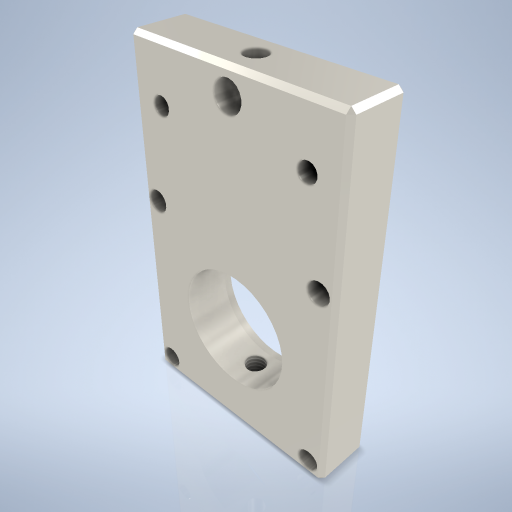
# Autodesk Inventor part: 01
Saved by Autodesk Inventor 2024.2 (Build 282272000, 272)
## iProperties
Created: 2024-05-15
Part Number: 01
Material: Titan
Document SubType Name: Modeling
Designer: Fabri
Density: 4.51 g/cm^3
Appearance: Titan
Author: Fabri
Autodesk Inventor part; units mm, degrees
note: some values were not read from the file. Chosen so that the rebuilt part matches the saved one: direction of "Bohrung1"; direction of "Bohrung3"; direction of "Bohrung4"; direction of "Bohrung5".
ref_plane "YZ Plane" through (0, 0, 0) normal (1, 0, 0) x (0, 1, 0)
ref_plane "XZ Plane" through (0, 0, 0) normal (0, 1, 0) x (-1, 0, 0)
ref_plane "XY Plane" through (0, 0, 0) normal (0, 0, 1) x (1, 0, 0)
sketch "Skizze1" plane through (0, 0, 0) normal (0, 1, 0) x (-1, 0, 0)
  line L0 (-25, 40) -> (25, 40)
  line L1 (25, 40) -> (25, -40)
  line L2 (25, -40) -> (-25, -40)
  line L3 (-25, -40) -> (-25, 40)
  line L4 (-25, 40) -> (25, -40) construction
  line L5 (25, 40) -> (-25, -40) construction
  point P0 (0, 0)
  dimension "d0" = 50
  dimension "d1" = 80
  constraints: 12 end point, 2 midpoint, 2 parallel, 1 horizontal, 1 perpendicular
  measures "d0" distance between parallel lines of L3 L1
  measures "d1" distance between parallel lines of L2 L0
extrude "Extrusion1" add sketch "Skizze1" along normal blind 13
sketch "Skizze2" plane through (0, 13, 0) normal (0, 1, 0) x (1, 0, 0)
  line L0 (25, 40) -> (-25, 40) projected
  point P0 (0, 0)
  point P1 (0, 15)
  dimension "d11" = 25
  constraints: 1 vertical alignment
  measures "d11" distance from line of L0 point (0, 15)
hole "Bohrung1" at (0, 13, -15) direction (0, -1, 0) diameter 27 depth 13 counterbore diameter 29 counterbore depth 2.5
sketch "Skizze3" plane through (0, 13, 0) normal (0, 1, 0) x (1, 0, 0)
  circle A0 centre (0, 15) radius 14.5 projected
  line L0 (25, 40) -> (-25, 40) projected
  line L1 (0, 40) -> (0, -45.4457) construction
  line L2 (25, -40) -> (25, 40) projected
  line L3 (25, 15) -> (-24, 15) construction
  point P0 (0, 0)
  point P1 (-21.124, -6.124)
  point P2 (-21.124, 36.124)
  point P3 (21.124, -6.124)
  point P4 (21.124, 36.124)
  dimension "d19" = 42.248
  dimension "d21" = 42.248
  dimension "d61" = 25
  constraints: 4 end point, 2 horizontal alignment, 2 symmetric about line, 2 vertical alignment, 1 horizontal, 1 midpoint, 1 point on line, 1 vertical
  measures "d19" distance of point (21.124, 36.124) point (21.124, -6.124)
  measures "d21" distance of point (-21.124, -6.124) point (21.124, -6.124)
  measures "d61" distance between parallel lines of L0 L3
hole "Bohrung2" at (-21.124, 13, 6.124) at (-21.124, 13, -36.124) at (21.124, 13, 6.124) at (21.124, 13, -36.124) direction (0, -1, 0) diameter 5 end through all
sketch "Skizze4" plane through (0, 13, 0) normal (0, 1, 0) x (1, 0, 0)
  point P0 (0, 0)
  point P1 (0, -34.4945)
  constraints: 1 vertical alignment
hole "Bohrung3" at (0, 13, 34.4945) direction (0, -1, 0) diameter 6.5 depth 13
sketch "Skizze5" plane through (0, 13, 0) normal (0, 1, 0) x (1, 0, 0)
  circle A0 centre (0, 15) radius 14.5 projected
  circle A1 centre (0, -34.4945) radius 3.25 projected
  line L0 (-25, -40) -> (25, -40) projected
  point P0 (0, 0)
  point P1 (-17.5, -27.5)
  point P2 (17.5, -27.5)
  dimension "d39" = 35
  dimension "d40" = 17.5
  dimension "d60" = 12.5
  constraints: 1 horizontal alignment
  measures "d39" distance of point (-17.5, -27.5) point (17.5, -27.5)
  measures "d40" horizontal distance of A1.centre point (17.5, -27.5)
  measures "d60" distance from line of L0 point (-17.5, -27.5)
hole "Bohrung4" at (-17.5, 13, 27.5) at (17.5, 13, 27.5) direction (0, -1, 0) diameter 4.134 depth 13 thread size "M5x0.8" class "6H" standard "ISO Metric profile"
sketch "Skizze6" plane through (25, 0, -40) normal (0, 0, -1) x (-1, 0, 0)
  line L0 (50, 0) -> (50, 13) projected
  line L1 (0, 0) -> (50, 0) projected
  point P0 (25, 0)
  point P1 (25, 6.5)
  point P2 (50, 6.5)
  point P3 (25, 0)
  constraints: 2 midpoint, 1 horizontal alignment, 1 vertical alignment
hole "Bohrung5" at (0, 6.5, -40) direction (0, 0, 1) diameter 4.917 depth 80 thread size "M6x1" class "6H" standard "ISO Metric profile"
sketch "Skizze7" plane through (-23, 0, -40) normal (0, 0, 1) x (1, 0, 0)
  line L0 (-2, 0) -> (-2, 13) projected
  line L1 (-2, 0) -> (48, 0) projected
  point P0 (23, 0)
  point P1 (4, 6.5)
  point P2 (42, 6.5)
  point P3 (-2, 6.5)
  point P4 (23, 0)
  point P5 (23, 0)
  dimension "d55" = 19
  dimension "d56" = 19
  constraints: 3 midpoint, 2 horizontal alignment
  measures "d55" horizontal distance of point (23, 0) point (4, 6.5)
  measures "d56" horizontal distance of point (23, 0) point (42, 6.5)
hole "Bohrung6" at (-19, 6.5, -40) at (19, 6.5, -40) direction (0, 0, 1) diameter 4.134 depth 14 thread size "M5x0.8" class "6H" standard "ISO Metric profile"
chamfer "Fasen1" distance 1 angle 45 12 edges at (25, 13, 0) (-25, 13, 0) (0, 13, 40) (0, 13, -40) (25, 0, 0) (0, 0, -40) (-25, 0, 0) (0, 0, 40) (-25, 6.5, 40) (-25, 6.5, -40) (25, 6.5, 40) (25, 6.5, -40)
equation "\"d19\" = d21"
